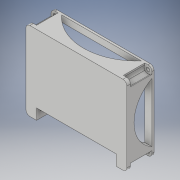
# Autodesk Inventor part: CyberDeckHDPower1
Saved by Autodesk Inventor 2019.4 (Build 234330000, 330)
## iProperties
Created: 2020-08-29
Part Number: CyberDeckHDPower1
Material: Generic
Document SubType Name: Modeling
Designer: Briti
Density: 1 g/cm^3
Appearance: Default
Author: Briti
## iProperties of the stored document _3DPrint.ipt
Created: 2020-08-29
Part Number: _3DPrint
Material: Generic
Document SubType Name: Modeling
Designer: Briti
Density: 1 g/cm^3
Appearance: Default
Author: Briti
Autodesk Inventor part; units mm, degrees
ref_plane "YZ Plane" through (0, 0, 0) normal (1, 0, 0) x (0, 1, 0)
ref_plane "XZ Plane" through (0, 0, 0) normal (0, 1, 0) x (-1, 0, 0)
ref_plane "XY Plane" through (0, 0, 0) normal (0, 0, 1) x (1, 0, 0)
sketch "Sketch1" plane through (0, 0, 0) normal (0, 0, 1) x (1, 0, 0)
  line L0 (-65, -49.5) -> (65, -49.5) construction
  line L1 (65, -49.5) -> (65, 49.5) construction
  line L2 (65, 49.5) -> (-65, 49.5) construction
  line L3 (-65, 49.5) -> (-65, -49.5) construction
  line L4 (-65, -49.5) -> (65, 49.5) construction
  line L5 (65, -49.5) -> (-65, 49.5) construction
  arc A0 (-65, 55) -> (-70.5, 49.5) centre (-65, 49.5) ccw
  arc A1 (70.5, 49.5) -> (65, 55) centre (65, 49.5) ccw
  arc A2 (65, -55) -> (70.5, -49.5) centre (65, -49.5) ccw
  arc A3 (-70.5, -49.5) -> (-65, -55) centre (-65, -49.5) ccw
  line L6 (-70.5, 49.5) -> (-70.5, -49.5)
  line L7 (-65, -55) -> (65, -55)
  line L8 (70.5, -49.5) -> (70.5, 49.5)
  line L9 (65, 55) -> (-65, 55)
  line L10 (-60.6244, -46.1678) -> (-60.6244, 46.1678)
  line L11 (-60.6244, 46.1678) -> (60.6244, 46.1678)
  line L12 (60.6244, 46.1678) -> (60.6244, -46.1678)
  line L13 (60.6244, -46.1678) -> (-60.6244, -46.1678)
  point P0 (0, 0)
  dimension "d0" = 130
  dimension "d1" = 99
  dimension "d2" = 11
  dimension "d3" = 11
  dimension "d4" = 11
  dimension "d5" = 11
  constraints: 28 end point, 8 point on circle, 5 tangent, 4 centre point, 4 coincident, 4 point on line, 3 perpendicular, 2 midpoint, 2 parallel, 1 horizontal, 1 vertical
  measures "d0" distance of L2.end L1.end
  measures "d1" distance of L1.end L0.end
  measures "d2" diameter of A0
  measures "d3" diameter of A1
  measures "d4" diameter of A2
  measures "d5" diameter of A3
extrude "Extrusion1" add sketch "Sketch1" along normal blind 3
sketch "Sketch2" plane through (0, 0, 3) normal (0, 0, 1) x (1, 0, 0)
  arc A0 (-65, 55) -> (-70.5, 49.5) centre (-65, 49.5) ccw projected
  circle A1 centre (-65, 49.5) radius 2.4
  arc A2 (70.5, 49.5) -> (65, 55) centre (65, 49.5) ccw projected
  circle A3 centre (65, 49.5) radius 2.4
  arc A4 (65, -55) -> (70.5, -49.5) centre (65, -49.5) ccw projected
  circle A5 centre (65, -49.5) radius 2.4
  arc A6 (-70.5, -49.5) -> (-65, -55) centre (-65, -49.5) ccw projected
  circle A7 centre (-65, -49.5) radius 2.4
  point P0 (0, 0)
  dimension "d8" = 4.8
  dimension "d9" = 4.8
  dimension "d10" = 4.8
  dimension "d11" = 4.8
  constraints: 4 centre point, 4 coincident
  measures "d8" diameter of A1
  measures "d9" diameter of A3
  measures "d10" diameter of A5
  measures "d11" diameter of A7
extrude "Extrusion2" cut sketch "Sketch2" against normal blind 8
sketch "Sketch3" plane through (0, 0, 3) normal (0, 0, 1) x (1, 0, 0)
  circle A0 centre (-65, 49.5) radius 2.4 construction
  circle A1 centre (-65, 49.5) radius 5.5 construction
  circle A2 centre (65, 49.5) radius 2.4 construction
  circle A3 centre (65, 49.5) radius 5.5 construction
  circle A4 centre (65, -49.5) radius 2.4 construction
  circle A5 centre (65, -49.5) radius 5.5 construction
  circle A6 centre (-65, -49.5) radius 2.4 construction
  circle A7 centre (-65, -49.5) radius 5.5 construction
  line L0 (-60.6244, -46.1678) -> (-60.6244, 46.1678) projected
  line L1 (-65, 55) -> (65, 55) projected
  line L2 (-60.6244, 52.8322) -> (-60.6244, 55)
  line L3 (-60.6244, 55) -> (60.6244, 55)
  line L4 (60.6244, 55) -> (60.6244, 52.8322)
  line L5 (60.6244, 46.1678) -> (-60.6244, 46.1678)
  arc A8 (-60.6244, 46.1678) -> (-60.6244, 52.8322) centre (-65, 49.5) ccw
  line L6 (60.6244, 46.1678) -> (-60.6244, 46.1678) projected
  arc A9 (60.6244, 52.8322) -> (60.6244, 46.1678) centre (65, 49.5) ccw
  line L7 (70.5, 49.5) -> (70.5, -49.5) projected
  line L8 (69.3756, 46.1678) -> (70.5, 46.1678)
  line L9 (70.5, 46.1678) -> (70.5, -46.1678)
  line L10 (70.5, -46.1678) -> (69.3756, -46.1678)
  line L11 (60.6244, -46.1678) -> (60.6244, 46.1678)
  arc A10 (69.3756, -46.1678) -> (60.6244, -46.1678) centre (65, -49.5) ccw
  arc A11 (60.6244, 46.1678) -> (69.3756, 46.1678) centre (65, 49.5) ccw
  line L12 (-70.5, -49.5) -> (-70.5, 49.5) projected
  line L13 (-69.3756, 46.1678) -> (-70.5, 46.1678)
  line L14 (-70.5, 46.1678) -> (-70.5, 41.1678)
  line L15 (-70.5, 41.1678) -> (-60.6244, 41.1678)
  line L16 (-60.6244, 41.1678) -> (-60.6244, 46.1678)
  arc A12 (-69.3756, 46.1678) -> (-60.6244, 46.1678) centre (-65, 49.5) ccw
  line L17 (-69.3756, -46.1678) -> (-70.5, -46.1678)
  line L18 (-70.5, -46.1678) -> (-70.5, -41.1678)
  line L19 (-70.5, -41.1678) -> (-60.6244, -41.1678)
  line L20 (-60.6244, -41.1678) -> (-60.6244, -46.1678)
  arc A13 (-60.6244, -46.1678) -> (-69.3756, -46.1678) centre (-65, -49.5) ccw
  line L21 (65, -55) -> (-65, -55) projected
  line L22 (-60.6244, -52.8322) -> (-60.6244, -55)
  line L23 (-60.6244, -55) -> (-55.6244, -55)
  line L24 (-55.6244, -55) -> (-55.6244, -46.1678)
  line L25 (-55.6244, -46.1678) -> (-60.6244, -46.1678)
  line L26 (-60.6244, -46.1678) -> (60.6244, -46.1678) projected
  arc A14 (-60.6244, -52.8322) -> (-60.6244, -46.1678) centre (-65, -49.5) ccw
  line L27 (60.6244, -52.8322) -> (60.6244, -55)
  line L28 (60.6244, -55) -> (55.6244, -55)
  line L29 (55.6244, -55) -> (55.6244, -46.1678)
  line L30 (55.6244, -46.1678) -> (60.6244, -46.1678)
  arc A15 (60.6244, -46.1678) -> (60.6244, -52.8322) centre (65, -49.5) ccw
  line L31 (-60.6244, 52.8322) -> (-60.6244, 55)
  arc A16 (60.6244, 46.1678) -> (69.3756, 46.1678) centre (65, 49.5) ccw
  line L32 (69.3756, 46.1678) -> (70.5, 46.1678)
  line L33 (70.5, 46.1678) -> (70.5, -46.1678)
  line L34 (70.5, -46.1678) -> (69.3756, -46.1678)
  arc A17 (69.3756, -46.1678) -> (60.6244, -46.1678) centre (65, -49.5) ccw
  line L35 (60.6244, -46.1678) -> (60.6244, 46.1678) projected
  line L36 (60.6244, -46.1678) -> (60.6244, 46.1678)
  arc A18 (60.6244, 52.8322) -> (60.6244, 46.1678) centre (65, 49.5) ccw
  line L37 (60.6244, 52.8322) -> (60.6244, 55)
  line L38 (60.6244, 55) -> (-60.6244, 55)
  line L39 (-60.6244, 55) -> (-60.6244, 52.8322)
  arc A19 (-60.6244, 46.1678) -> (-60.6244, 52.8322) centre (-65, 49.5) ccw
  line L40 (-60.6244, 46.1678) -> (60.6244, 46.1678)
  line L41 (-60.6244, 46.1678) -> (-60.6244, 41.1678)
  line L42 (-60.6244, 41.1678) -> (-70.5, 41.1678)
  line L43 (-70.5, 41.1678) -> (-70.5, 46.1678)
  line L44 (-70.5, 46.1678) -> (-69.3756, 46.1678)
  arc A20 (-69.3756, 46.1678) -> (-60.6244, 46.1678) centre (-65, 49.5) ccw
  arc A21 (-60.6244, -46.1678) -> (-69.3756, -46.1678) centre (-65, -49.5) ccw
  line L45 (-60.6244, -46.1678) -> (-60.6244, -41.1678)
  line L46 (-60.6244, -41.1678) -> (-70.5, -41.1678)
  line L47 (-70.5, -41.1678) -> (-70.5, -46.1678)
  line L48 (-70.5, -46.1678) -> (-69.3756, -46.1678)
  line L49 (-60.6244, -46.1678) -> (-55.6244, -46.1678)
  line L50 (-55.6244, -46.1678) -> (-55.6244, -55)
  line L51 (-55.6244, -55) -> (-60.6244, -55)
  line L52 (-60.6244, -55) -> (-60.6244, -52.8322)
  arc A22 (-60.6244, -52.8322) -> (-60.6244, -46.1678) centre (-65, -49.5) ccw
  point P0 (0, 0)
  dimension "d14" = 5
  dimension "d15" = 5
  dimension "d16" = 5
  dimension "d17" = 5
  constraints: 90 end point, 38 point on circle, 19 centre point, 19 concentric, 15 perpendicular, 14 collinear, 12 parallel, 6 point on line, 4 coincident, 2 horizontal, 2 vertical
  measures "d14" distance of L14.end L13.end
  measures "d15" distance of L17.end L18.end
  measures "d16" distance of L23.end L22.end
  measures "d17" distance of L27.end L28.end
extrude "Extrusion3" add sketch "Sketch3" along normal blind 30 contours A13 L17 L12 L19 L0 | L25 L24 L21 L22 A14 | L15 L12 L13 A12 L0 | L26 A15 L27 L21 L29 | A8 L2 L1 L4 A9 L5 | L11 A11 L8 L7 L10 A10
sketch "Sketch4" plane through (-65, 55, 0) normal (0, 1, 0) x (1, 0, 0)
  line L0 (125.6244, -33) -> (4.3756, -33) construction
  line L1 (65, -33) -> (65, -28) construction
  line L2 (124.5, -3) -> (125.6244, -3) construction
  line L3 (125.6244, -3) -> (120.6244, -3) construction
  line L4 (-5.5, -3) -> (4.3756, -3) construction
  line L5 (120.6244, -3) -> (9.3756, -3) construction
  line L6 (4.3756, -3) -> (9.3756, -3) construction
  arc A0 (9.3756, -3) -> (120.6244, -3) centre (65, 46.3814) ccw
  line L7 (9.3756, -3) -> (9.3756, -33) projected
  line L8 (120.6244, -3) -> (9.3756, -3)
  point P0 (65, 0)
  dimension "d20" = 5
  dimension "d21" = 5
  constraints: 8 end point, 3 point on circle, 1 centre point, 1 collinear, 1 horizontal, 1 midpoint, 1 perpendicular, 1 vertical
  measures "d20" distance of L1.start L1.end
  measures "d21" distance of L2.end L3.end
extrude "Extrusion4" cut sketch "Sketch4" against normal blind 10
sketch "Sketch5" plane through (70.5, -49.5, 0) normal (1, 0, 0) x (0, 0, -1)
  line L0 (-33, 95.6678) -> (-33, 3.3322) construction
  line L1 (-33, 49.5) -> (-28, 49.5) construction
  line L2 (0, 3.3322) -> (-3, 3.3322) construction
  line L3 (-3, 8.3322) -> (-3, 90.6678) construction
  line L4 (-3, 3.3322) -> (-3, 8.3322) construction
  line L5 (-3, 95.6678) -> (-33, 95.6678) construction
  line L6 (-3, 95.6678) -> (-3, 90.6678) construction
  line L7 (-3, 90.6678) -> (-33, 90.6678) projected
  arc A0 (-3, 90.6678) -> (-3, 8.3322) centre (18.3957, 49.5) ccw
  line L8 (-3, 8.3322) -> (-3, 90.6678)
  point P0 (0, 49.5)
  dimension "d24" = 5
  constraints: 8 end point, 3 collinear, 3 point on circle, 1 centre point, 1 horizontal, 1 midpoint
  measures "d24" distance of L1.start L1.end
extrude "Extrusion5" cut sketch "Sketch5" against normal blind 10
sketch "Sketch6" plane through (0, 0, 33) normal (0, 0, 1) x (1, 0, 0)
  line L0 (70.5, 46.1678) -> (70.5, 49.5) construction
  line L1 (70.5, 46.1678) -> (70.5, 59.6838) construction
  line L2 (-65, -55) -> (65, -55)
  line L3 (70.5, -49.5) -> (70.5, 49.5)
  line L4 (65, 55) -> (-65, 55)
  line L5 (-70.5, 49.5) -> (-70.5, -49.5)
  line L6 (-70.5, -55) -> (70.5, 55) construction
  line L7 (70.5, -55) -> (-70.5, 55) construction
  arc A0 (-65, 55) -> (-70.5, 49.5) centre (-65, 49.5) ccw projected
  arc A1 (-65, 55) -> (-70.5, 49.5) centre (-65, 49.5) ccw
  line L8 (-70.5, -49.5) -> (-70.5, 49.5) projected
  arc A2 (-70.5, -49.5) -> (-65, -55) centre (-65, -49.5) ccw projected
  arc A3 (-70.5, -49.5) -> (-65, -55) centre (-65, -49.5) ccw
  arc A4 (65, -55) -> (70.5, -49.5) centre (65, -49.5) ccw projected
  arc A5 (65, -55) -> (70.5, -49.5) centre (65, -49.5) ccw
  arc A6 (70.5, 49.5) -> (65, 55) centre (65, 49.5) ccw projected
  arc A7 (70.5, 49.5) -> (65, 55) centre (65, 49.5) ccw
  point P0 (0, 0)
  constraints: 16 point on circle, 14 end point, 4 centre point, 2 midpoint, 2 parallel, 2 point on line, 1 horizontal, 1 perpendicular, 1 vertical
extrude "Extrusion6" add sketch "Sketch6" along normal blind 5
sketch "Sketch7" plane through (0, 0, 38) normal (0, 0, 1) x (1, 0, 0)
  line L0 (55.6244, -46.1678) -> (55.6244, -55) projected
  line L1 (55.6244, -55) -> (55.6244, -40)
  line L2 (55.6244, -40) -> (-55.6244, -40)
  line L3 (-55.6244, -40) -> (-55.6244, -55)
  line L4 (-55.6244, -55) -> (55.6244, -55)
  point P0 (0, 0)
  dimension "d29" = 15
  constraints: 8 end point, 2 parallel, 1 collinear, 1 perpendicular
  measures "d29" distance of L0.end L1.end
extrude "Extrusion7" cut sketch "Sketch7" against normal blind 5
body "Solid1"
